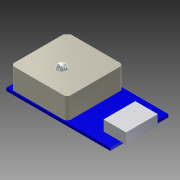
# Autodesk Inventor part: MediatekMT3329
Saved by Autodesk Inventor 2012 (Build 160160000, 160)
## iProperties
Created: 2012-05-21
Part Number: MediatekMT3329
Material: Default
Document SubType Name: Modeling
Designer: x02s
Density: 1 g/cm^3
Author: x02s
Autodesk Inventor part; units mm, degrees
ref_plane "YZ Plane" through (0, 0, 0) normal (1, 0, 0) x (0, 1, 0)
ref_plane "XZ Plane" through (0, 0, 0) normal (0, 1, 0) x (-1, 0, 0)
ref_plane "XY Plane" through (0, 0, 0) normal (0, 0, 1) x (1, 0, 0)
sketch "Sketch1" plane through (0, 0, 0) normal (0, 0, 1) x (1, 0, 0)
  line L0 (0, 8.25) -> (-29.5, 8.25)
  line L1 (-29.5, 8.25) -> (-29.5, -8.25)
  line L2 (-29.5, -8.25) -> (0, -8.25)
  line L3 (0, -8.25) -> (0, 8.25)
  circle A0 centre (-20.5, 0) radius 1.5
  point P0 (0, 0)
  point P1 (0, 0)
  dimension "d0" = 16.5
  dimension "d1" = 29.5
  dimension "d2" = 3
  dimension "d3" = 20.5
  constraints: 8 end point, 2 parallel, 1 centre point, 1 coincident, 1 horizontal, 1 horizontal alignment, 1 midpoint, 1 perpendicular
  measures "d0" distance of L2.end L0.start
  measures "d1" distance of L0.start L0.end
  measures "d2" diameter of A0
  measures "d3" distance from line of L3 A0.centre
extrude "Extrusion1" add sketch "Sketch1" along normal blind 0.8
sketch "Sketch2" plane through (0, 0, 0.8) normal (0, 0, 1) x (1, 0, 0)
  line L0 (-28.5, 8) -> (-12.5, 8)
  line L1 (-12.5, 8) -> (-12.5, -8)
  line L2 (-12.5, -8) -> (-28.5, -8)
  line L3 (-28.5, -8) -> (-28.5, 8)
  line L4 (0, 8.25) -> (0, -8.25) projected
  line L5 (-29.5, 8.25) -> (-29.5, -8.25) projected
  circle A0 centre (-20.5, 0) radius 1.5 projected
  point P0 (0, 0)
  point P1 (-12.5, 0)
  point P2 (0, 0)
  dimension "d6" = 16
  dimension "d7" = 16
  dimension "d8" = 1
  constraints: 8 end point, 2 midpoint, 2 parallel, 1 horizontal, 1 horizontal alignment, 1 perpendicular
  measures "d6" distance of L0.start L0.end
  measures "d7" distance of L2.end L0.start
  measures "d8" distance between parallel lines of L5 L3
extrude "Extrusion2" add sketch "Sketch2" along normal blind 6 contours L0 L1 L2 L3 | A0
fillet "Fillet1" radius 1 3 edges at (-12.5, -8, 3.8) (-12.5, 8, 3.8) (-28.5, -8, 3.8)
chamfer "Chamfer1" distance 1 angle 45 1 edges at (-28.5, 8, 3.8)
sketch "Sketch3" plane through (0, 0, 0.8) normal (0, 0, 1) x (1, 0, 0)
  line L0 (-4.9, 3.75) -> (1.5, 3.75)
  line L1 (1.5, 3.75) -> (1.5, -5.25)
  line L2 (1.5, -5.25) -> (-4.9, -5.25)
  line L3 (-4.9, -5.25) -> (-4.9, 3.75)
  line L4 (0, -8.25) -> (-29.5, -8.25) projected
  line L5 (0, -8.25) -> (0, 8.25) projected
  point P0 (0, 0)
  dimension "d15" = 9
  dimension "d16" = 3
  dimension "d17" = 6.4
  dimension "d18" = 1.5
  constraints: 8 end point, 2 parallel, 1 horizontal, 1 perpendicular
  measures "d15" distance of L0.end L1.end
  measures "d16" distance between parallel lines of L4 L2
  measures "d17" distance between parallel lines of L1 L3
  measures "d18" distance between parallel lines of L5 L1
extrude "Extrusion3" add sketch "Sketch3" along normal blind 3
sketch "Sketch4" plane through (0, 0, 6.8) normal (0, 0, 1) x (1, 0, 0)
  circle A0 centre (-20.5, -1.5) radius 1.25
  line L0 (-13.5, -8) -> (-27.5, -8) projected
  line L1 (-12.5, 7) -> (-12.5, -7) projected
  point P0 (0, 0)
  dimension "d21" = 2.5
  dimension "d22" = 6.5
  dimension "d23" = 8
  constraints: 1 centre point
  measures "d21" diameter of A0
  measures "d22" distance from line of L0 A0.centre
  measures "d23" distance from line of L1 A0.centre
extrude "Extrusion4" add sketch "Sketch4" along normal blind 1
fillet "Fillet2" radius 1 1 edges at (-21.75, -1.5, 7.8)
sketch "Sketch5" plane through (0, 0, 0) normal (0, 0, -1) x (-1, 0, 0)
  line L0 (0, -8.25) -> (0, 8.25) projected
  line L1 (0, 8.25) -> (29.5, 8.25) projected
  line L2 (29.5, -8.25) -> (0, -8.25) projected
  line L3 (0.5, 6.6) -> (4, 6.6)
  line L4 (4, 6.6) -> (4, 4.6)
  line L5 (4, 4.6) -> (0.5, 4.6)
  line L6 (0.5, 4.6) -> (0.5, 6.6)
  line L7 (0.5, 3.8) -> (4, 3.8)
  line L8 (4, 3.8) -> (4, 1.8)
  line L9 (4, 1.8) -> (0.5, 1.8)
  line L10 (0.5, 1.8) -> (0.5, 3.8)
  line L11 (0.5, 1) -> (4, 1)
  line L12 (4, 1) -> (4, -1)
  line L13 (4, -1) -> (0.5, -1)
  line L14 (0.5, -1) -> (0.5, 1)
  line L15 (0.5, -1.8) -> (4, -1.8)
  line L16 (4, -1.8) -> (4, -3.8)
  line L17 (4, -3.8) -> (0.5, -3.8)
  line L18 (0.5, -3.8) -> (0.5, -1.8)
  line L19 (0.5, -4.6) -> (4, -4.6)
  line L20 (4, -4.6) -> (4, -6.6)
  line L21 (4, -6.6) -> (0.5, -6.6)
  line L22 (0.5, -6.6) -> (0.5, -4.6)
  line L23 (4.5, 6.75) -> (10.6136, 6.75) construction
  line L24 (10.6136, 6.75) -> (10.6136, -8.25) construction
  line L25 (10.6136, -8.25) -> (4.5, -8.25) construction
  line L26 (4.5, -8.25) -> (4.5, 6.75) construction
  spline S0 degree 2 poles (5.2804, 5.1941) (5.1212, 5.1941) (4.8574, 5.2913) (4.7626, 5.3898) knots 0 0 0 1 2 2 2
  spline S1 degree 2 poles (4.7626, 5.3898) (4.6677, 5.4895) (4.5669, 5.7836) (4.5669, 5.9745) knots 0 0 0 1 2 2 2
  spline S2 degree 2 poles (4.5669, 5.9745) (4.5669, 6.1556) (4.669, 6.4425) (4.7638, 6.5446) knots 0 0 0 1 2 2 2
  spline S3 degree 2 poles (4.7638, 6.5446) (4.8549, 6.643) (5.1224, 6.75) (5.2816, 6.75) knots 0 0 0 1 2 2 2
  spline S4 degree 2 poles (5.2816, 6.75) (5.3582, 6.75) (5.4968, 6.7281) (5.56, 6.7087) knots 0 0 0 1 2 2 2
  spline S5 degree 2 poles (5.56, 6.7087) (5.611, 6.6941) (5.735, 6.6406) (5.7727, 6.6212) knots 0 0 0 1 2 2 2
  line L27 (5.7727, 6.6212) -> (5.7727, 6.3805)
  line L28 (5.7727, 6.3805) -> (5.7557, 6.3805)
  spline S6 degree 2 poles (5.7557, 6.3805) (5.718, 6.4133) (5.639, 6.4729) (5.566, 6.5069) knots 0 0 0 1 2 2 2
  spline S7 degree 2 poles (5.566, 6.5069) (5.5053, 6.5373) (5.3485, 6.5774) (5.2585, 6.5774) knots 0 0 0 1 2 2 2
  spline S8 degree 2 poles (5.2585, 6.5774) (5.0421, 6.5774) (4.7747, 6.2516) (4.7747, 5.9806) knots 0 0 0 1 2 2 2
  spline S9 degree 2 poles (4.7747, 5.9806) (4.7747, 5.8298) (4.8452, 5.6037) (4.9121, 5.5259) knots 0 0 0 1 2 2 2
  spline S10 degree 2 poles (4.9121, 5.5259) (4.9765, 5.4481) (5.1588, 5.3667) (5.2731, 5.3667) knots 0 0 0 1 2 2 2
  spline S11 degree 2 poles (5.2731, 5.3667) (5.357, 5.3667) (5.5247, 5.391) (5.5818, 5.4153) knots 0 0 0 1 2 2 2
  line L29 (5.5818, 5.4153) -> (5.5818, 5.8031)
  line L30 (5.5818, 5.8031) -> (5.2342, 5.8031)
  line L31 (5.2342, 5.8031) -> (5.2342, 5.9781)
  line L32 (5.2342, 5.9781) -> (5.7788, 5.9781)
  line L33 (5.7788, 5.9781) -> (5.7788, 5.3229)
  spline S12 degree 2 poles (5.7788, 5.3229) (5.7411, 5.3059) (5.6122, 5.2536) (5.5575, 5.2378) knots 0 0 0 1 2 2 2
  spline S13 degree 2 poles (5.5575, 5.2378) (5.4834, 5.216) (5.3643, 5.1941) (5.2804, 5.1941) knots 0 0 0 1 2 2 2
  line L34 (7.1025, 5.2233) -> (6.8788, 5.2233)
  line L35 (6.8788, 5.2233) -> (6.2152, 6.5166)
  line L36 (6.2152, 6.5166) -> (6.2152, 5.2233)
  line L37 (6.2152, 5.2233) -> (6.0292, 5.2233)
  line L38 (6.0292, 5.2233) -> (6.0292, 6.7233)
  line L39 (6.0292, 6.7233) -> (6.3124, 6.7233)
  line L40 (6.3124, 6.7233) -> (6.9165, 5.5357)
  line L41 (6.9165, 5.5357) -> (6.9165, 6.7233)
  line L42 (6.9165, 6.7233) -> (7.1025, 6.7233)
  line L43 (7.1025, 6.7233) -> (7.1025, 5.2233)
  spline S14 degree 2 poles (8.5891, 5.972) (8.5891, 5.7666) (8.4226, 5.436) (8.2828, 5.3436) knots 0 0 0 1 2 2 2
  spline S15 degree 2 poles (8.2828, 5.3436) (8.1686, 5.2719) (7.934, 5.2233) (7.7516, 5.2233) knots 0 0 0 1 2 2 2
  line L44 (7.7516, 5.2233) -> (7.4064, 5.2233)
  line L45 (7.4064, 5.2233) -> (7.4064, 6.7233)
  line L46 (7.4064, 6.7233) -> (7.748, 6.7233)
  spline S16 degree 2 poles (7.748, 6.7233) (7.9595, 6.7233) (8.2002, 6.66) (8.2853, 6.6041) knots 0 0 0 1 2 2 2
  spline S17 degree 2 poles (8.2853, 6.6041) (8.4299, 6.5081) (8.5891, 6.1908) (8.5891, 5.972) knots 0 0 0 1 2 2 2
  spline S18 degree 2 poles (8.3813, 5.9745) (8.3813, 6.1471) (8.267, 6.3914) (8.154, 6.4607) knots 0 0 0 1 2 2 2
  spline S19 degree 2 poles (8.154, 6.4607) (8.0737, 6.5081) (7.8926, 6.5506) (7.7577, 6.5506) knots 0 0 0 1 2 2 2
  line L47 (7.7577, 6.5506) -> (7.6058, 6.5506)
  line L48 (7.6058, 6.5506) -> (7.6058, 5.3959)
  line L49 (7.6058, 5.3959) -> (7.7577, 5.3959)
  spline S20 degree 2 poles (7.7577, 5.3959) (7.8902, 5.3959) (8.0908, 5.4384) (8.1722, 5.4955) knots 0 0 0 1 2 2 2
  spline S21 degree 2 poles (8.1722, 5.4955) (8.2767, 5.566) (8.3813, 5.7994) (8.3813, 5.9745) knots 0 0 0 1 2 2 2
  spline S22 degree 2 poles (5.5186, 2.6998) (5.5186, 2.5916) (5.4494, 2.4068) (5.3861, 2.3387) knots 0 0 0 1 2 2 2
  spline S23 degree 2 poles (5.3861, 2.3387) (5.3229, 2.2707) (5.1345, 2.1917) (5.0178, 2.1917) knots 0 0 0 1 2 2 2
  spline S24 degree 2 poles (5.0178, 2.1917) (4.9109, 2.1917) (4.7018, 2.2391) (4.6252, 2.2767) knots 0 0 0 1 2 2 2
  line L50 (4.6252, 2.2767) -> (4.6252, 2.4895)
  line L51 (4.6252, 2.4895) -> (4.6398, 2.4895)
  spline S25 degree 2 poles (4.6398, 2.4895) (4.6629, 2.4724) (4.7492, 2.4287) (4.8015, 2.4092) knots 0 0 0 1 2 2 2
  spline S26 degree 2 poles (4.8015, 2.4092) (4.861, 2.3886) (4.9595, 2.3655) (5.0215, 2.3655) knots 0 0 0 1 2 2 2
  spline S27 degree 2 poles (5.0215, 2.3655) (5.0823, 2.3655) (5.1965, 2.4092) (5.2378, 2.4566) knots 0 0 0 1 2 2 2
  spline S28 degree 2 poles (5.2378, 2.4566) (5.2755, 2.5016) (5.3144, 2.6207) (5.3144, 2.701) knots 0 0 0 1 2 2 2
  spline S29 degree 2 poles (5.3144, 2.701) (5.3144, 2.7812) (5.2707, 2.8833) (5.2293, 2.9173) knots 0 0 0 1 2 2 2
  spline S30 degree 2 poles (5.2293, 2.9173) (5.1868, 2.955) (5.0604, 2.9866) (4.9838, 2.9866) knots 0 0 0 1 2 2 2
  spline S31 degree 2 poles (4.9838, 2.9866) (4.9011, 2.9866) (4.737, 2.9611) (4.6872, 2.9502) knots 0 0 0 1 2 2 2
  line L52 (4.6872, 2.9502) -> (4.6872, 3.7233)
  line L53 (4.6872, 3.7233) -> (5.5101, 3.7233)
  line L54 (5.5101, 3.7233) -> (5.5101, 3.547)
  line L55 (5.5101, 3.547) -> (4.8805, 3.547)
  line L56 (4.8805, 3.547) -> (4.8805, 3.1471)
  spline S32 degree 2 poles (4.8805, 3.1471) (4.9169, 3.1519) (4.9874, 3.1556) (5.0166, 3.1556) knots 0 0 0 1 2 2 2
  spline S33 degree 2 poles (5.0166, 3.1556) (5.1321, 3.1556) (5.2913, 3.1179) (5.3643, 3.062) knots 0 0 0 1 2 2 2
  spline S34 degree 2 poles (5.3643, 3.062) (5.4384, 3.0061) (5.5186, 2.8359) (5.5186, 2.6998) knots 0 0 0 1 2 2 2
  line L57 (6.8655, 3.7233) -> (6.3489, 2.2233)
  line L58 (6.3489, 2.2233) -> (6.1337, 2.2233)
  line L59 (6.1337, 2.2233) -> (5.6171, 3.7233)
  line L60 (5.6171, 3.7233) -> (5.831, 3.7233)
  line L61 (5.831, 3.7233) -> (6.2468, 2.4773)
  line L62 (6.2468, 2.4773) -> (6.6625, 3.7233)
  line L63 (6.6625, 3.7233) -> (6.8655, 3.7233)
  spline S35 degree 2 poles (5.7131, 0.5519) (5.7982, 0.4522) (5.893, 0.1605) (5.893, -0.0267) knots 0 0 0 1 2 2 2
  spline S36 degree 2 poles (5.893, -0.0267) (5.893, -0.2091) (5.8006, -0.5045) (5.7131, -0.6041) knots 0 0 0 1 2 2 2
  spline S37 degree 2 poles (5.7131, -0.6041) (5.6207, -0.7087) (5.3764, -0.8083) (5.2293, -0.8083) knots 0 0 0 1 2 2 2
  spline S38 degree 2 poles (5.2293, -0.8083) (5.0774, -0.8083) (4.8343, -0.705) (4.7455, -0.6041) knots 0 0 0 1 2 2 2
  spline S39 degree 2 poles (4.7455, -0.6041) (4.6592, -0.5045) (4.5669, -0.2115) (4.5669, -0.0267) knots 0 0 0 1 2 2 2
  spline S40 degree 2 poles (4.5669, -0.0267) (4.5669, 0.1617) (4.6605, 0.4485) (4.7468, 0.5519) knots 0 0 0 1 2 2 2
  spline S41 degree 2 poles (4.7468, 0.5519) (4.8343, 0.6515) (5.0786, 0.7549) (5.2293, 0.7549) knots 0 0 0 1 2 2 2
  spline S42 degree 2 poles (5.2293, 0.7549) (5.3825, 0.7549) (5.628, 0.6479) (5.7131, 0.5519) knots 0 0 0 1 2 2 2
  spline S43 degree 2 poles (5.6852, -0.0267) (5.6852, 0.1216) (5.6207, 0.3513) (5.5624, 0.4267) knots 0 0 0 1 2 2 2
  spline S44 degree 2 poles (5.5624, 0.4267) (5.5028, 0.5045) (5.3351, 0.5823) (5.2306, 0.5823) knots 0 0 0 1 2 2 2
  spline S45 degree 2 poles (5.2306, 0.5823) (5.1224, 0.5823) (4.9595, 0.5069) (4.8975, 0.4267) knots 0 0 0 1 2 2 2
  spline S46 degree 2 poles (4.8975, 0.4267) (4.8379, 0.3501) (4.7747, 0.1191) (4.7747, -0.0267) knots 0 0 0 1 2 2 2
  spline S47 degree 2 poles (4.7747, -0.0267) (4.7747, -0.3221) (5.0227, -0.6357) (5.2306, -0.6357) knots 0 0 0 1 2 2 2
  spline S48 degree 2 poles (5.2306, -0.6357) (5.4384, -0.6357) (5.6852, -0.3221) (5.6852, -0.0267) knots 0 0 0 1 2 2 2
  spline S49 degree 2 poles (6.6357, -0.8083) (6.5032, -0.8083) (6.3063, -0.7391) (6.237, -0.6698) knots 0 0 0 1 2 2 2
  spline S50 degree 2 poles (6.237, -0.6698) (6.158, -0.592) (6.0936, -0.3732) (6.0936, -0.2127) knots 0 0 0 1 2 2 2
  line L64 (6.0936, -0.2127) -> (6.0936, 0.7233)
  line L65 (6.0936, 0.7233) -> (6.2929, 0.7233)
  line L66 (6.2929, 0.7233) -> (6.2929, -0.2127)
  spline S51 degree 2 poles (6.2929, -0.2127) (6.2929, -0.3173) (6.3197, -0.4583) (6.3574, -0.5154) knots 0 0 0 1 2 2 2
  spline S52 degree 2 poles (6.3574, -0.5154) (6.3975, -0.5762) (6.5361, -0.6382) (6.6357, -0.6382) knots 0 0 0 1 2 2 2
  spline S53 degree 2 poles (6.6357, -0.6382) (6.7293, -0.6382) (6.8752, -0.5762) (6.9153, -0.5154) knots 0 0 0 1 2 2 2
  spline S54 degree 2 poles (6.9153, -0.5154) (6.953, -0.4583) (6.9797, -0.3185) (6.9797, -0.2176) knots 0 0 0 1 2 2 2
  line L67 (6.9797, -0.2176) -> (6.9797, 0.7233)
  line L68 (6.9797, 0.7233) -> (7.1791, 0.7233)
  line L69 (7.1791, 0.7233) -> (7.1791, -0.2127)
  spline S55 degree 2 poles (7.1791, -0.2127) (7.1791, -0.3695) (7.1159, -0.5932) (7.0357, -0.6698) knots 0 0 0 1 2 2 2
  spline S56 degree 2 poles (7.0357, -0.6698) (6.9639, -0.7403) (6.7743, -0.8083) (6.6357, -0.8083) knots 0 0 0 1 2 2 2
  line L70 (7.8148, -0.7767) -> (7.8148, 0.5458)
  line L71 (7.8148, 0.5458) -> (7.3116, 0.5458)
  line L72 (7.3116, 0.5458) -> (7.3116, 0.7233)
  line L73 (7.3116, 0.7233) -> (8.5174, 0.7233)
  line L74 (8.5174, 0.7233) -> (8.5174, 0.5458)
  line L75 (8.5174, 0.5458) -> (8.0142, 0.5458)
  line L76 (8.0142, 0.5458) -> (8.0142, -0.7767)
  line L77 (8.0142, -0.7767) -> (7.8148, -0.7767)
  line L78 (5.1746, -3.7767) -> (4.5936, -3.7767)
  line L79 (4.5936, -3.7767) -> (4.5936, -3.6236)
  line L80 (4.5936, -3.6236) -> (4.7844, -3.6236)
  line L81 (4.7844, -3.6236) -> (4.7844, -2.4299)
  line L82 (4.7844, -2.4299) -> (4.5936, -2.4299)
  line L83 (4.5936, -2.4299) -> (4.5936, -2.2767)
  line L84 (4.5936, -2.2767) -> (5.1746, -2.2767)
  line L85 (5.1746, -2.2767) -> (5.1746, -2.4299)
  line L86 (5.1746, -2.4299) -> (4.9838, -2.4299)
  line L87 (4.9838, -2.4299) -> (4.9838, -3.6236)
  line L88 (4.9838, -3.6236) -> (5.1746, -3.6236)
  line L89 (5.1746, -3.6236) -> (5.1746, -3.7767)
  line L90 (6.4947, -3.7767) -> (6.2711, -3.7767)
  line L91 (6.2711, -3.7767) -> (5.6074, -2.4834)
  line L92 (5.6074, -2.4834) -> (5.6074, -3.7767)
  line L93 (5.6074, -3.7767) -> (5.4214, -3.7767)
  line L94 (5.4214, -3.7767) -> (5.4214, -2.2767)
  line L95 (5.4214, -2.2767) -> (5.7046, -2.2767)
  line L96 (5.7046, -2.2767) -> (6.3088, -3.4643)
  line L97 (6.3088, -3.4643) -> (6.3088, -2.2767)
  line L98 (6.3088, -2.2767) -> (6.4947, -2.2767)
  line L99 (6.4947, -2.2767) -> (6.4947, -3.7767)
  line L100 (4.6519, -6.7767) -> (4.6519, -5.2767)
  line L101 (4.6519, -5.2767) -> (5.5904, -5.2767)
  line L102 (5.5904, -5.2767) -> (5.5904, -5.4542)
  line L103 (5.5904, -5.4542) -> (4.8513, -5.4542)
  line L104 (4.8513, -5.4542) -> (4.8513, -5.8651)
  line L105 (4.8513, -5.8651) -> (5.5405, -5.8651)
  line L106 (5.5405, -5.8651) -> (5.5405, -6.0425)
  line L107 (5.5405, -6.0425) -> (4.8513, -6.0425)
  line L108 (4.8513, -6.0425) -> (4.8513, -6.5993)
  line L109 (4.8513, -6.5993) -> (5.5904, -6.5993)
  line L110 (5.5904, -6.5993) -> (5.5904, -6.7767)
  line L111 (5.5904, -6.7767) -> (4.6519, -6.7767)
  line L112 (6.8825, -6.7767) -> (6.6588, -6.7767)
  line L113 (6.6588, -6.7767) -> (5.9951, -5.4834)
  line L114 (5.9951, -5.4834) -> (5.9951, -6.7767)
  line L115 (5.9951, -6.7767) -> (5.8092, -6.7767)
  line L116 (5.8092, -6.7767) -> (5.8092, -5.2767)
  line L117 (5.8092, -5.2767) -> (6.0924, -5.2767)
  line L118 (6.0924, -5.2767) -> (6.6965, -6.4643)
  line L119 (6.6965, -6.4643) -> (6.6965, -5.2767)
  line L120 (6.6965, -5.2767) -> (6.8825, -5.2767)
  line L121 (6.8825, -5.2767) -> (6.8825, -6.7767)
  point P0 (0, 0)
  dimension "d27" = 0.5
  dimension "d28" = 3.5
  dimension "d29" = 2
  dimension "d30" = 0.8
  dimension "d31" = 0.8
  dimension "d32" = 0.8
  dimension "d33" = 0.8
  dimension "d34" = 1.65
  dimension "d35" = 1.65
  dimension "d36" = 0.5
  dimension "d37" = 1.5
  constraints: 40 end point, 12 collinear, 10 parallel, 5 horizontal, 5 perpendicular, 1 point on line, 2 other
  measures "d27" distance between parallel lines of L0 L6
  measures "d28" distance of L3.start L3.end
  measures "d29" distance of L3.end L4.end
  measures "d30" distance between parallel lines of L7 L5
  measures "d31" distance between parallel lines of L11 L9
  measures "d32" distance between parallel lines of L15 L13
  measures "d33" distance between parallel lines of L19 L17
  measures "d34" distance between parallel lines of L21 L2
  measures "d35" distance between parallel lines of L1 L3
  measures "d36" distance between parallel lines of L4 L26
  measures "d37" distance between parallel lines of L1 L23
extrude "Extrusion5" add sketch "Sketch5" along normal blind 0.1
equation "\"d7\" = d6"
equation "\"d31\" = d30"
equation "\"d32\" = d31"
equation "\"d33\" = d32"
equation "\"d34\" = d35"
body "Solid1"
